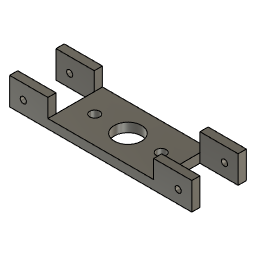
Z_cap (Autodesk Fusion 360 design; units mm, degrees)
Autodesk Fusion 360 part; units mm, degrees
sketch "Sketch1" plane through (0, 0, 0) normal (0, 0, 1) x (1, 0, 0)
  line L0 (0, 0) -> (30, 0)
  line L1 (30, 0) -> (30, 30)
  line L2 (30, 30) -> (0, 30)
  line L3 (0, 30) -> (0, 0)
  line L4 (0, 30) -> (30, 30)
  line L5 (30, 30) -> (30, 25.5)
  line L6 (30, 25.5) -> (0, 25.5)
  line L7 (0, 25.5) -> (0, 30)
  line L8 (0, 0) -> (30, 0)
  line L9 (30, 0) -> (30, 4.5)
  line L10 (30, 4.5) -> (0, 4.5)
  line L11 (0, 4.5) -> (0, 0)
  line L12 (25.1749, 0) -> (83.1749, 0)
  line L13 (83.1749, 0) -> (83.1749, 30)
  line L14 (83.1749, 30) -> (25.1749, 30)
  line L15 (25.1749, 30) -> (25.1749, 0)
  line L16 (83.1749, 30) -> (87.6749, 30)
  line L17 (87.6749, 30) -> (87.6749, 0)
  line L18 (87.6749, 0) -> (83.1749, 0)
  line L19 (83.1749, 0) -> (83.1749, 30)
  line L20 (83.1749, 30) -> (108.1749, 30)
  line L21 (108.1749, 30) -> (108.1749, 25.5)
  line L22 (108.1749, 25.5) -> (83.1749, 25.5)
  line L23 (83.1749, 25.5) -> (83.1749, 30)
  line L24 (83.1749, 0) -> (108.1749, 0)
  line L25 (108.1749, 0) -> (108.1749, 4.5)
  line L26 (108.1749, 4.5) -> (83.1749, 4.5)
  line L27 (83.1749, 4.5) -> (83.1749, 0)
  dimension "d1" = 30
  dimension "d2" = 30
  dimension "d3" = 4.5
  dimension "d4" = 4.5
  dimension "d5" = 58
  dimension "d6" = 30
  dimension "d8" = 4.5
  dimension "d9" = 30
  dimension "d10" = 25
  dimension "d11" = 4.5
  dimension "d12" = 25
  dimension "d13" = 4.5
  constraint horizontal L0
  constraint vertical L1
  constraint horizontal L2
  constraint vertical L3
  constraint coincident L0.start L3.end
  constraint horizontal L4
  constraint vertical L5
  constraint horizontal L6
  constraint vertical L7
  constraint horizontal L8
  constraint vertical L9
  constraint horizontal L10
  constraint vertical L11
  constraint horizontal L12
  constraint vertical L13
  constraint horizontal L14
  constraint vertical L15
  constraint coincident L8 L12.start
  constraint horizontal L16
  constraint vertical L17
  constraint horizontal L18
  constraint vertical L19
  constraint horizontal L20
  constraint vertical L21
  constraint horizontal L22
  constraint vertical L23
  constraint horizontal L24
  constraint vertical L25
  constraint horizontal L26
  constraint vertical L27
  measures "d1" distance of L0.start L0.end
  measures "d2" distance of L0.start L2.end
  measures "d3" distance of L2.end L6.end
  measures "d4" distance of L0.start L10.end
  measures "d5" distance of L12.start L12.end
  measures "d6" distance of L12.start L14.end
  measures "d8" distance of L13.end L16.end
  measures "d9" distance of L13.end L12.end
  measures "d10" distance of L13.end L20.end
  measures "d11" distance of L13.end L22.end
  measures "d12" distance of L12.end L24.end
  measures "d13" distance of L12.end L26.end
extrude "Extrude1" add sketch "Sketch1" along normal blind 15 contours L0 L3 L8 L10 L11 L15 | L2 L3 L4 L6 L7 L15 | L13 L17 L18 L19 L24 L26 L27 | L17 L24 L25 L26 | L13 L16 L17 L19 L20 L22 L23 | L17 L20 L21 L22 makes body 1 at (16.7833, 25.5, 5) makes body 2 at (91.5082, 30, 5) makes body 3 at (16.7833, 4.5, 5) makes body 4 at (99.8415, 0, 5)
sketch "Sketch2" plane through (0, 0, 0) normal (0, 0, -1) x (1, 0, 0)
  line L0 (108.1749, -25.5) -> (83.1749, -25.5)
  line L1 (83.1749, -25.5) -> (83.1749, -30)
  line L2 (83.1749, -30) -> (108.1749, -30)
  line L3 (108.1749, -30) -> (108.1749, -25.5)
  line L4 (24.987, -0.0649) -> (83.1749, -0.0649)
  line L5 (83.1749, -0.0649) -> (83.1749, -30)
  line L6 (83.1749, -30) -> (24.987, -30)
  line L7 (24.987, -30) -> (24.987, -0.0649)
  constraint horizontal L4
  constraint vertical L5
  constraint horizontal L6
  constraint vertical L7
  constraint coincident L1.end L2.start
extrude "Extrude2" add sketch "Sketch2" against normal blind 5 contours L1 L4 L5 L6 L7 bodies 1 2 3 4
extrude "Extrude3" cut 2 faces at (0, 28.5, 5) (0, 3, 5) along direction (1, 0, 0) blind 0.175 on bodies 1 bodies 1
extrude "Extrude4" cut 1 faces at (24.987, 18.5, 1.6667) along direction (1, 0, 0) up to surface (0.1879 mm away) on bodies 1 bodies 1
extrude "Extrude5" cut 1 faces at (99.8415, 0, 5) along direction (0, 1, 0) up to surface (0.0649 mm away) on bodies 1 bodies 1
extrude "Extrude6" cut 1 faces at (8.5083, 0, 5) along direction (0, 1, 0) up to surface (0.0649 mm away) on bodies 1 bodies 1
sketch "Sketch3" plane through (0, 0, 5) normal (0, 0, 1) x (-1, 0, 0)
  line L0 (-25.1749, -25.5) -> (-25.1749, -4.5)
  line L1 (-25.1749, -4.5) -> (-25.1749, -0.0649)
  line L2 (-25.1749, -0.0649) -> (-83.1749, -0.0649)
  line L3 (-83.1749, -0.0649) -> (-83.1749, -4.5)
  line L4 (-83.1749, -4.5) -> (-83.1749, -25.5)
  line L5 (-83.1749, -25.5) -> (-83.1749, -30)
  line L6 (-83.1749, -30) -> (-25.1749, -30)
  line L7 (-25.1749, -30) -> (-25.1749, -25.5)
  point P0 (-54.1749, -15)
  dimension "d27" = 29
  dimension "d28" = 28
  dimension "d29" = 15
  dimension "d30" = 14.9351
  measures "d27" distance of L0 P0
  measures "d29" distance of L6 P0
  measures "d30" distance of L2 P0
hole "Hole1" at (54.1749, 15, 5) direction (0, 0, -1) diameter 15 depth 15 tip angle 118 bodies 1
sketch "Sketch4" plane through (0, 0, 5) normal (0, 0, 1) x (-1, 0, 0)
  circle A0 centre (-54.1749, -15) radius 7.5
  line L0 (-25.1749, -25.5) -> (-25.1749, -4.5)
  line L1 (-25.1749, -4.5) -> (-25.1749, -0.0649)
  line L2 (-25.1749, -0.0649) -> (-83.1749, -0.0649)
  line L3 (-83.1749, -0.0649) -> (-83.1749, -4.5)
  line L4 (-83.1749, -4.5) -> (-83.1749, -25.5)
  line L5 (-83.1749, -25.5) -> (-83.1749, -30)
  line L6 (-83.1749, -30) -> (-25.1749, -30)
  line L7 (-25.1749, -30) -> (-25.1749, -25.5)
  point P0 (-72.4249, -15)
  point P1 (-35.9249, -15)
  dimension "d34" = 18.25
  dimension "d35" = 18.25
  dimension "d36" = 15
  dimension "d37" = 15
  measures "d34" horizontal distance of A0.centre P0
  measures "d35" horizontal distance of A0.centre P1
  measures "d36" distance of L6 P0
  measures "d37" distance of L6 P1
hole "Hole2" at (35.9249, 15, 5) at (72.4249, 15, 5) direction (0, 0, -1) diameter 5.5 depth 15 tip angle 118 bodies 1
extrude "Extrude7" add 2 faces at (0.175, 28.5, 5) (0.175, 3.0216, 5) along direction (-1, 0, 0) blind 1 on bodies 1 bodies 1
extrude "Extrude8" add 2 faces at (108.1749, 28.5, 5) (108.1749, 1.5433, 5) along direction (1, 0, 0) blind 1 on bodies 1 bodies 1
sketch "Sketch5" plane through (0, 30, 0) normal (0, 1, 0) x (-1, 0, 0)
  line L0 (0.825, 15) -> (-25.1749, 15)
  line L1 (-25.1749, 15) -> (-25.1749, 5)
  line L2 (-25.1749, 5) -> (-83.1749, 5)
  line L3 (-83.1749, 5) -> (-83.1749, 15)
  line L4 (-83.1749, 15) -> (-109.1749, 15)
  line L5 (-109.1749, 15) -> (-109.1749, 0)
  line L6 (-109.1749, 0) -> (0.825, 0)
  line L7 (0.825, 0) -> (0.825, 15)
  point P0 (-9.175, 4)
  point P1 (-9.175, 11)
  dimension "d45" = 4
  dimension "d46" = 4
  dimension "d47" = 10
  dimension "d48" = 10
  dimension "d49" = 7
  measures "d45" distance of L0 P1
  measures "d46" distance of L6 P0
  measures "d47" distance of L7 P1
  measures "d48" distance of L7 P0
  measures "d49" distance of P0 P1
hole "Hole3" at (9.175, 30, 11) at (9.175, 30, 4) direction (0, -1, 0) diameter 3.2 depth 200 tip angle 118 bodies 1
sketch "Sketch6" plane through (0, 30, 0) normal (0, 1, 0) x (-1, 0, 0)
  circle A0 centre (-9.175, 11) radius 1.6
  circle A1 centre (-9.175, 4) radius 1.6
  line L0 (0.825, 15) -> (-25.1749, 15)
  line L1 (-25.1749, 15) -> (-25.1749, 5)
  line L2 (-25.1749, 5) -> (-83.1749, 5)
  line L3 (-83.1749, 5) -> (-83.1749, 15)
  line L4 (-83.1749, 15) -> (-109.1749, 15)
  line L5 (-109.1749, 15) -> (-109.1749, 0)
  line L6 (-109.1749, 0) -> (0.825, 0)
  line L7 (0.825, 0) -> (0.825, 15)
  point P0 (-99.1749, 11)
  point P1 (-99.1749, 4)
  dimension "d53" = 10
  dimension "d54" = 10
  dimension "d55" = 4
  dimension "d56" = 4
  measures "d53" distance of L5 P0
  measures "d54" distance of L5 P1
  measures "d55" distance of L6 P1
  measures "d56" distance of L4 P0
hole "Hole4" at (99.1749, 30, 11) at (99.1749, 30, 4) direction (0, -1, 0) diameter 3.2 depth 200 tip angle 118 bodies 1
delete_face "DeleteFace1" 1 faces at (99.9401, 1.5433, 2.5948) on bodies 1
delete_face "DeleteFace2" 1 faces at (99.0951, 1.5433, 12.598) on bodies 1
delete_face "DeleteFace3" 1 faces at (99.9401, 28.5, 2.5948) on bodies 1
delete_face "DeleteFace4" 1 faces at (99.0156, 28.5, 12.592) on bodies 1
delete_face "DeleteFace5" 4 faces at (9.2548, 3.0216, 5.598) (9.2548, 3.0216, 12.598) (9.2548, 28.5, 5.598) (9.2548, 28.5, 12.598) on bodies 1
extrude "Extrude9" cut 2 faces at (109.1749, 28.5, 5) (109.1749, 1.5433, 5) along direction (-1, 0, 0) blind 4 on bodies 1 bodies 1
extrude "Extrude10" cut 2 faces at (-0.825, 28.5, 5) (-0.825, 3.0216, 5) along direction (1, 0, 0) blind 4 on bodies 1 bodies 1
extrude "Extrude11" cut 1 faces at (3.175, 3.0216, 5) along direction (1, 0, 0) blind 1 on bodies 1 bodies 1
extrude "Extrude12" cut 1 faces at (3.175, 28.5, 5) along direction (1, 0, 0) blind 1 on bodies 1 bodies 1
extrude "Extrude13" cut 2 faces at (105.1749, 1.5433, 5) (105.1749, 28.5, 5) along direction (-1, 0, 0) blind 1 on bodies 1 bodies 1
sketch "Sketch7" plane through (0, 30, 0) normal (0, 1, 0) x (-1, 0, 0)
  line L0 (-104.1749, 15) -> (-104.1749, 0)
  line L1 (-104.1749, 0) -> (-4.175, 0)
  line L2 (-4.175, 0) -> (-4.175, 15)
  line L3 (-4.175, 15) -> (-25.1749, 15)
  line L4 (-25.1749, 15) -> (-25.1749, 5)
  line L5 (-25.1749, 5) -> (-83.1749, 5)
  line L6 (-83.1749, 5) -> (-83.1749, 15)
  line L7 (-83.1749, 15) -> (-104.1749, 15)
  point P0 (-96.675, 7)
  point P1 (-11.675, 7)
  dimension "d70" = 85
  dimension "d71" = 7
  dimension "d72" = 7
  dimension "d73" = 7.5
  dimension "d74" = 8.9999
  measures "d70" distance of P0 P1
  measures "d71" distance of L1 P0
  measures "d72" distance of L1 P1
  measures "d73" distance of L2 P1
hole "Hole5" at (96.675, 30, 7) at (11.675, 30, 7) direction (0, -1, 0) diameter 3.4 depth 10000 tip angle 118 bodies 1
